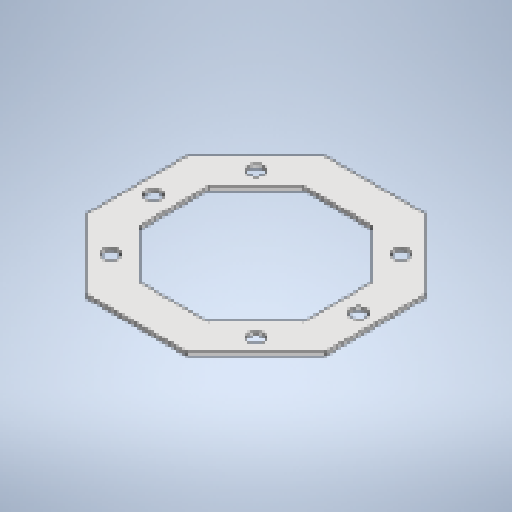
# Autodesk Inventor part: DSB 110 drain sustem flange
Saved by Autodesk Inventor 2025.1 (Build 291241020, 241B)
## iProperties
Created: 2024-12-09
Part Number: DSB 110 drain sustem flange
Material: Stainless Steel
Document SubType Name: Sheet Metal
Designer: admin
Mass: 1674.72 g
Surface Area: 927.524 cm^2
Volume: 209.34 cm^3
Density: 8 g/cm^3
Flat Pattern Width: 28 cm
Flat Pattern Length: 28 cm
Flat Pattern Area: 784 cm^2
Sheet Metal Rule: AISI304 4mm Die 32
Sheet Metal Width: 280.000 mm
Sheet Metal Length: 280.000 mm
Sheet Metal Area: 78400.000 mm^2
Appearance: Default
Octaeder_side: 80.000 mm
Octaeder_flange_lenth: 43.431 mm
Author: user
Autodesk Inventor part; units mm, degrees
ref_plane "YZ Plane" through (0, 0, 0) normal (1, 0, 0) x (0, 1, 0)
ref_plane "XZ Plane" through (0, 0, 0) normal (0, 1, 0) x (-1, 0, 0)
ref_plane "XY Plane" through (0, 0, 0) normal (0, 0, 1) x (1, 0, 0)
sketch "Sketch1" plane through (0, 0, 0) normal (0, 0, 1) x (1, 0, 0)
  circle A0 centre (0, 0) radius 96.5685 construction
  circle A1 centre (0, 0) radius 140 construction
  line L0 (140, -140) -> (-140, -140)
  line L1 (-140, -140) -> (-140, 140)
  line L2 (-140, 140) -> (140, 140)
  line L3 (140, 140) -> (140, -140)
  line L4 (140, -140) -> (-140, 140) construction
  line L5 (-140, -140) -> (140, 140) construction
  line L6 (57.9899, 140) -> (140, 57.9899)
  line L7 (140, 57.9899) -> (140, -57.9899)
  line L8 (140, -57.9899) -> (57.9899, -140)
  line L9 (57.9899, -140) -> (-57.9899, -140)
  line L10 (-57.9899, -140) -> (-140, -57.9899)
  line L11 (-140, -57.9899) -> (-140, 57.9899)
  line L12 (-140, 57.9899) -> (-57.9899, 140)
  line L13 (-57.9899, 140) -> (57.9899, 140)
  line L14 (40, 96.5685) -> (96.5685, 40)
  line L15 (96.5685, 40) -> (96.5685, -40)
  line L16 (96.5685, -40) -> (40, -96.5685)
  line L17 (40, -96.5685) -> (-40, -96.5685)
  line L18 (-40, -96.5685) -> (-96.5685, -40)
  line L19 (-96.5685, -40) -> (-96.5685, 40)
  line L20 (-96.5685, 40) -> (-40, 96.5685)
  line L21 (-40, 96.5685) -> (40, 96.5685)
  point P0 (0, 140)
  point P1 (-57.9899, 140)
  point P2 (-140, 57.9899)
  point P3 (-140, -57.9899)
  point P4 (-57.9899, -140)
  point P5 (57.9899, -140)
  point P6 (140, -57.9899)
  point P7 (140, 57.9899)
  point P8 (57.9899, 140)
  point P9 (0, 96.5685)
  point P10 (0, 140)
  dimension "d23" = 280
  dimension "d41" = 80
  dimension "d42" = 43.4315
  measures "d41" distance of L17.end L18.end
  measures "d42" distance of point (0, 96.569) point (0, 140)
extrude "Plate1" add sketch "Sketch1" along normal blind 4 contours L0 L10 L1 L12 L2 L6 L3 L8
sketch "Sketch6" plane through (0, 0, 0) normal (0, 0, 1) x (1, 0, 0)
  line L0 (0, 0) -> (0, 120) construction
  circle A0 centre (0, 0) radius 120 construction
  line L1 (0, 0) -> (84.8528, 84.8528) construction
  circle A1 centre (84.8528, 84.8528) radius 9
  dimension "d32" = 18
  dimension "d33" = 240
  dimension "d34" = 45
  constraints: 4 end point, 2 centre point, 2 coincident, 2 point on circle, 1 vertical
  measures "d32" diameter of A1
  measures "d33" diameter of A0
  measures "d34" angle of L0 L1
extrude "Cut2" cut sketch "Sketch6" along normal blind 4
pattern_circular "Circular Pattern2" count 3 over 90 about axis through (0, 0, -10) along (0, 0, -1) of "Cut2"
mirror "Mirror1" about plane through (0, 0, 0) normal (1, 0, 0) of "Cut2", "Circular Pattern2"
equation "\"d23\" = Flange_D_outer"
equation "\"d32\" = Flange_d_hole_diam"
equation "\"d33\" = Flange_D1_hole_center"
equation "\"d35\" = Thickness"
equation "\"d2\" = Thickness"
equation "\"BendReliefWidth\" = Thickness"
equation "\"BendReliefDepth\" = 0.5 * Thickness"
equation "\"CornerReliefSize\" = 4 * Thickness"
equation "\"MinimumRemnant\" = 2 * Thickness"
equation "\"TransitionRadius\" = BendRadius"
equation "\"JacobiRadiusSize\" = BendRadius"
equation "\"GapSize\" = Thickness"
equation "\"Octaeder_flange_lenth\" = d42"
equation "\"Flange_D_outer\" = 280"
equation "\"Flange_d_hole_diam\" = 18"
equation "\"Flange_D1_hole_center\" = 240"
equation "\"Thickness\" = 4"
equation "\"BendRadius\" = 6"
body "Solid1"
